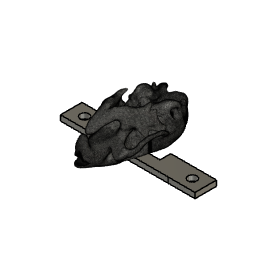
Headbar_notch (Autodesk Fusion 360 design; units mm, degrees)
Autodesk Fusion 360 part; units mm, degrees
sketch "Sketch1" plane through (0, 0, 0) normal (0, 0, 1) x (1, 0, 0)
  line L0 (-47.100252, 10.15177) -> (-22.100252, 10.15177)
  line L1 (-22.100252, 10.15177) -> (-22.100252, 6.15177)
  line L2 (-22.100252, 6.15177) -> (-47.100252, 6.15177)
  line L3 (-47.100252, 6.15177) -> (-47.100252, 10.15177)
  circle A0 centre (-44.600252, 8.15177) radius 0.825
  circle A1 centre (-24.600252, 8.169598) radius 0.825
  line L4 (-47.100252, 8.15177) -> (-44.600252, 8.15177) construction
  line L5 (-22.100252, 8.15177) -> (-24.600252, 8.169598)
  dimension "d1" = 25
  dimension "d2" = 4
  dimension "d3" = 1.65
  dimension "d4" = 1.65
  dimension "d7" = 2.5
  dimension "d8" = 2.5
  constraint horizontal L0
  constraint vertical L1
  constraint horizontal L2
  constraint vertical L3
  constraint perpendicular L3 L4
  measures "d3" diameter of A0
  measures "d4" diameter of A1
extrude "Extrude1" add sketch "Sketch1" along normal blind 1
sketch "Sketch2" plane through (0, 6.15177, 0) normal (0, -1, 0) x (1, 0, 0)
  line L0 (-47.100252, 0) -> (-22.100252, 0)
  line L1 (-22.100252, 0) -> (-22.100252, 1)
  line L2 (-22.100252, 1) -> (-47.100252, 1)
  line L3 (-47.100252, 1) -> (-47.100252, 0)
  line L4 (-47.100252, 0.5) -> (-42.100252, 0.5) construction
  line L5 (-42.100252, 1) -> (-27.100252, 1)
  line L6 (-27.100252, 1) -> (-27.100252, 0)
  line L7 (-27.100252, 0) -> (-42.100252, 0)
  line L8 (-42.100252, 0) -> (-42.100252, 1)
  dimension "d9" = 5
  dimension "d10" = 15
  constraint perpendicular L3 L4
  constraint horizontal L5
  constraint vertical L6
  constraint horizontal L7
  constraint vertical L8
extrude "Extrude2" add sketch "Sketch2" along normal blind 0.0001 contours L0 L2 L5 L6 L7 L8 picked at (-32.100252, 0.666667)
sketch "Sketch3" plane through (0, 0, 0) normal (0, 0, -1) x (1, 0, 0)
  circle A0 centre (-24.600252, -8.169598) radius 0.825
  circle A1 centre (-44.600252, -8.15177) radius 0.825
  line L0 (-22.100252, -6.15177) -> (-27.100252, -6.15177)
  line L1 (-27.100252, -6.15177) -> (-27.100252, -6.15167)
  line L2 (-27.100252, -6.15167) -> (-42.100252, -6.15167)
  line L3 (-42.100252, -6.15167) -> (-42.100252, -6.15177)
  line L4 (-42.100252, -6.15177) -> (-47.100252, -6.15177)
  line L5 (-47.100252, -6.15177) -> (-47.100252, -10.15177)
  line L6 (-47.100252, -10.15177) -> (-22.100252, -10.15177)
  line L7 (-22.100252, -10.15177) -> (-22.100252, -6.15177)
  line L8 (-47.100252, -8.15177) -> (-40.100252, -8.15177) construction
  line L9 (-42.100252, -6.15177) -> (-40.100252, -6.15177) construction
  line L10 (-40.100252, -6.15177) -> (-29.100252, -6.15177)
  line L11 (-29.100252, -6.15177) -> (-29.100252, -10.15177)
  line L12 (-29.100252, -10.15177) -> (-40.100252, -10.15177)
  line L13 (-40.100252, -10.15177) -> (-40.100252, -6.15177)
  dimension "d13" = 7
  dimension "d14" = 2
  dimension "d15" = 11
  constraint perpendicular L5 L8
  constraint perpendicular L3 L9
  constraint horizontal L10
  constraint vertical L11
  constraint horizontal L12
  constraint vertical L13
extrude "Extrude3" cut sketch "Sketch3" against normal blind 1 contours L2 L6 L10 L11 L12 L13 picked at (-36.433585, -7.48507)
other "Base Mesh Feature1" in component "MeshBody1"
other "Modify1" in component "MeshBody1"
move_face "OffsetFaces1" offset 1.5 1 faces at (-29.100252, 7.485103, 0.333333)
move_face "OffsetFaces2" offset 1.5 1 faces at (-40.100252, 8.818407, 0.333333)
move_face "OffsetFaces3" offset 2 1 faces at (-33.266918, 6.151729, 0.333333)
component "MeshBody1" placed x (1, 0, 0) y (0, 1, 0) z (0, 0, 1) at (0, 0, 0)
